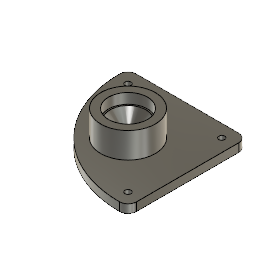
gear-bearing-holder (Autodesk Fusion 360 design; units mm, degrees)
Autodesk Fusion 360 part; units mm, degrees
sketch "Sketch1" plane through (0, 0, 0) normal (0, 0, 1) x (1, 0, 0)
  line L0 (0, 0) -> (70, 0)
  line L1 (70, 0) -> (70, 70)
  line L2 (70, 70) -> (0, 70)
  line L3 (0, 70) -> (0, 0)
  circle A0 centre (7.5, 62.5) radius 1.75
  circle A1 centre (62.5, 62.5) radius 1.75
  circle A2 centre (7.5, 7.5) radius 1.75
  circle A3 centre (62.5, 7.5) radius 1.75
  dimension "d1" = 70
  dimension "d2" = 70
  dimension "d3" = 3.5
  dimension "d4" = 7.5
  dimension "d5" = 7.5
  dimension "d8" = 55
  dimension "d9" = -55
  measures "d1" distance of L0.start L2.end
  measures "d2" distance of L0.start L0.end
  measures "d3" diameter of A0
  measures "d4" distance of L3 A0.centre
  measures "d5" distance of L2 A0.centre
extrude "Extrude1" add sketch "Sketch1" along normal blind 5
sketch "Sketch2" plane through (0, 0, 5) normal (0, 0, 1) x (-1, 0, 0)
  circle A0 centre (-62.5, -7.5) radius 1.75
  circle A1 centre (-7.5, -62.5) radius 1.75
  circle A2 centre (-7.5, -7.5) radius 1.75
  circle A3 centre (-62.5, -62.5) radius 1.75
  line L0 (0, -70) -> (0, 0)
  line L1 (0, 0) -> (-70, 0)
  line L2 (-70, 0) -> (-70, -70)
  line L3 (-70, -70) -> (0, -70)
  circle A4 centre (-35, -35) radius 11.4
  dimension "d12" = 22.8
  measures "d12" diameter of A4
extrude "Extrude2" cut sketch "Sketch2" against normal blind 5 contours A4
sketch "Sketch3" plane through (0, 0, 5) normal (0, 0, 1) x (-1, 0, 0)
  circle A0 centre (-35, -35) radius 11.4
  circle A1 centre (-62.5, -7.5) radius 1.75
  circle A2 centre (-7.5, -62.5) radius 1.75
  circle A3 centre (-7.5, -7.5) radius 1.75
  circle A4 centre (-62.5, -62.5) radius 1.75
  line L0 (0, -70) -> (0, 0)
  line L1 (0, 0) -> (-70, 0)
  line L2 (-70, 0) -> (-70, -70)
  line L3 (-70, -70) -> (0, -70)
  circle A5 centre (-35, -35) radius 16
  dimension "d15" = 32
  measures "d15" diameter of A5
extrude "Extrude3" add sketch "Sketch3" along normal blind 15 contours A0 | A5
sketch "Sketch4" plane through (0, 0, 20) normal (0, 0, 1) x (-1, 0, 0)
  circle A0 centre (-35, -35) radius 16
  circle A1 centre (-35, -35) radius 4.5
  dimension "d18" = 9
  measures "d18" diameter of A1
extrude "Extrude4" cut sketch "Sketch4" against normal blind 45 contours A1
sketch "Sketch5" plane through (0, 0, 20) normal (0, 0, 1) x (-1, 0, 0)
  circle A0 centre (-35, -35) radius 4.5
  circle A1 centre (-35, -35) radius 16
  circle A2 centre (-35, -35) radius 11.4
  dimension "d21" = 22.8
  measures "d21" diameter of A2
extrude "Extrude5" cut sketch "Sketch5" against normal blind 6 contours A2
extrude "Extrude6" add 1 faces at (25.9592, 35.7899, 5) along direction (0, 0, -1) blind 3.5
chamfer "Chamfer1" distance 6 angle 45 2 edges at (39.1955, 36.6273, 14) (39.1955, 36.6273, 1.5)
fillet "Fillet2" radius 65 1 edges at (0, 0, 2.5)
fillet "Fillet3" radius 5 3 edges at (70, 0, 2.5) (70, 70, 2.5) (0, 70, 2.5)
